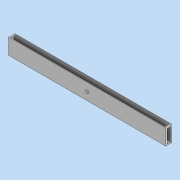
# Autodesk Inventor part: hashi1shado
Saved by Autodesk Inventor 2022 (Build 260153000, 153)
## iProperties
Created: 2024-05-14
Part Number: hashi1shado
Material: 一般
Document SubType Name: Modeling
Designer: ktamu
Density: 1 g/cm^3
Appearance: 既定
Author: ktamu
Autodesk Inventor part; units mm, degrees
ref_plane "YZ Plane" through (0, 0, 0) normal (1, 0, 0) x (0, 1, 0)
ref_plane "XZ Plane" through (0, 0, 0) normal (0, 1, 0) x (-1, 0, 0)
ref_plane "XY Plane" through (0, 0, 0) normal (0, 0, 1) x (1, 0, 0)
sketch "スケッチ2" plane through (0, 0, 0) normal (1, 0, 0) x (0, 1, 0)
  line L0 (25, 10) -> (-25, 10)
  line L1 (-25, 10) -> (-25, -10)
  line L2 (-25, -10) -> (25, -10)
  line L3 (25, -10) -> (25, 10)
  line L4 (25, 10) -> (-25, -10) construction
  line L5 (-25, 10) -> (25, -10) construction
  point P0 (0, 0)
  dimension "d4" = 50
  dimension "d5" = 20
  constraints: 12 end point, 2 midpoint, 2 parallel, 1 horizontal, 1 perpendicular
  measures "d4" distance of L2.end L1.end
  measures "d5" distance of L1.end L0.end
extrude "押し出し2" add sketch "スケッチ2" along normal mid plane 500
sketch "スケッチ3" plane through (-250, -25, 10) normal (0, 0, 1) x (1, 0, 0)
  circle A0 centre (250, 25) radius 5
  dimension "d8" = 10
  constraints: 1 centre point, 1 coincident
  measures "d8" diameter of A0
extrude "押し出し3" add sketch "スケッチ3" along normal blind 2
fillet "フィレット1" radius 2 2 edges at (250, 0, -10) (-250, 0, -10)
sketch "スケッチ4" plane through (250, 0, 0) normal (1, 0, 0) x (0, 0, -1)
  line L0 (-6, 21) -> (6, 21)
  line L1 (6, 21) -> (6, -21)
  line L2 (6, -21) -> (-6, -21)
  line L3 (-6, -21) -> (-6, 21)
  line L4 (-6, 21) -> (6, -21) construction
  line L5 (6, 21) -> (-6, -21) construction
  point P0 (0, 0)
  dimension "d12" = 12
  dimension "d13" = 42
  constraints: 12 end point, 2 midpoint, 2 parallel, 1 horizontal, 1 perpendicular
  measures "d12" distance of L1.end L2.end
  measures "d13" distance of L0.end L1.end
extrude "押し出し4" cut sketch "スケッチ4" against normal through all
sketch "スケッチ6" plane through (-250, -25, 10) normal (0, -1, 0) x (1, 0, 0)
  line L0 (4, -2) -> (496, -2)
  line L1 (496, -2) -> (496, -18)
  line L2 (496, -18) -> (4, -18)
  line L3 (4, -18) -> (4, -2)
  line L4 (4, -2) -> (496, -18) construction
  line L5 (496, -2) -> (4, -18) construction
  point P0 (250, -10)
  dimension "d16" = 492
  dimension "d17" = 16
  constraints: 12 end point, 2 midpoint, 2 parallel, 1 horizontal, 1 perpendicular
  measures "d16" distance of L1.end L2.end
  measures "d17" distance of L0.end L1.end
extrude "押し出し5" cut sketch "スケッチ6" against normal through all
